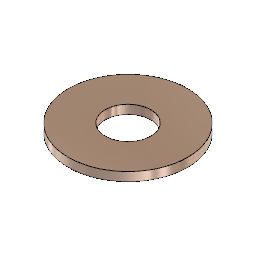
SHVFeedthroughFilterWithPulseLine_LEGEND60 (Autodesk Fusion 360 archive; units mm, degrees)
design "Washer"
Autodesk Fusion 360 part; units mm, degrees
sketch "Sketch1" plane through (0, 0, 0) normal (0, 0, 1) x (1, 0, 0)
  circle A0 centre (0, 0) radius 8.5
  circle A1 centre (0, 0) radius 3.2385
  dimension "d1" = 17
  dimension "d2" = 6.477
  constraint coincident A0.centre A1.centre
  measures "d1" diameter of A0
  measures "d2" diameter of A1
extrude "Extrude1" add sketch "Sketch1" along normal blind 1.27
sketch "Sketch2" plane through (0, 0, 0) normal (0, 0, -1) x (1, 0, 0)
  arc A0 (-2.7777, 8.0333) -> (2.7777, 8.0333) centre (0, 15) ccw
  circle A1 centre (0, 0) radius 8.5
  line L0 (0, -1.75) -> (0, -22.5)
  dimension "d6" = 15
  dimension "d10" = 7.5
  constraint coincident A0.end A1
  constraint coincident A0.start A1
  constraint coincident A0.centre L0
  measures "d6" distance of A1.centre A0.centre
  measures "d10" radius of A0
extrude "Extrude2" [rolled back] taper angle 0
pattern_circular "C-Pattern1" [rolled back] total angle 360

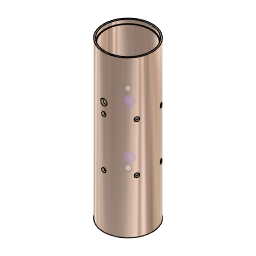
design "OuterTube"
Autodesk Fusion 360 part; units mm, degrees
sketch "Sketch1" plane through (0, 0, 0) normal (0, 0, 1) x (1, 0, 0)
  circle A0 centre (0, 0) radius 9.525
  circle A1 centre (0, 0) radius 8.7122
  dimension "d1" = 19.05
  dimension "d2" = 0.8128
  constraint coincident A0.centre A1.centre
  constraint concentric A0 A1
  measures "d1" diameter of A0
  measures "d2" distance of A0 A1
extrude "Extrude1" add sketch "Sketch1" along normal blind 76
sketch "Sketch2" plane through (0, 0, 0) normal (1, 0, 0) x (0, 1, 0)
  line L0 (0, 1.75) -> (0, 22.5)
  point P0 (0, 8)
  dimension "d8" = 8
  constraint coincident P0 L0
  measures "d8" distance of origin P0
hole "Hole1" at (0, 0, 8) direction (-1, 0, 0) diameter 2.3813 depth 30 tip angle 118
sketch "Sketch3" plane through (0, 0, 0) normal (0, 1, 0) x (1, 0, 0)
  point P0 (0, -36)
  dimension "d9" = 36
  measures "d9" distance of origin P0
hole "Hole2" at (0, 0, 36) direction (0, -1, 0) diameter 1.5875 depth 20 tip angle 118
pattern_circular "C-Pattern1" count 6 over 360 about axis through (0, 0, 1.75) along (0, 0, 1) of "Hole2"
sketch "Sketch4" plane through (0, 0, 0) normal (0, 0, -1) x (1, 0, 0)
  circle A0 centre (0, 0) radius 8.7122
  circle A1 centre (0, 0) radius 9.525
  circle A2 centre (0, 0) radius 9
  dimension "d15" = 18
  constraint coincident A0.centre A1.centre
  measures "d15" diameter of A2
extrude "Extrude2" cut sketch "Sketch4" against normal blind 1.5 contours A2
sketch "Sketch5" plane through (0, 0, 76) normal (0, 0, 1) x (-1, 0, 0)
  circle A0 centre (0, 0) radius 8.7122
  circle A1 centre (0, 0) radius 9.525
  circle A2 centre (0, 0) radius 9
  dimension "d18" = 18
  constraint concentric A0 A2
  measures "d18" diameter of A2
extrude "Extrude3" cut sketch "Sketch5" against normal blind 1.5 contours A2
sketch "Sketch7" plane through (0, 0, 0) normal (0, 1, 0) x (1, 0, 0)
  line L0 (9.525, 0) -> (-9.525, 0)
  line L1 (-9.525, -76) -> (9.525, -76)
  point P0 (0, -55)
  dimension "d42" = 21
  measures "d42" distance of P0 L1
hole "Hole4" at (0, 0, 55) direction (0, -1, 0) diameter 1.5875 end through all
pattern_circular "C-Pattern2" count 6 over 360 about axis through (0, 0, 1.75) along (0, 0, 1) of "Hole4"
sketch "Sketch8" plane through (0, 0, 0) normal (0, 0, -1) x (1, 0, 0)
  circle A0 centre (0, 0) radius 9
  circle A1 centre (0, 0) radius 9.525
  line L0 (7.064, 5.5449) -> (8.334, 3.3451)
  line L1 (8.334, 3.3451) -> (-7.064, -5.5449)
  line L2 (-7.064, -5.5449) -> (-8.334, -3.3451)
  line L3 (-8.334, -3.3451) -> (7.064, 5.5449)
  line L4 (1.75, 0) -> (22.5, 0)
  line L5 (0, -1.75) -> (0, -22.5)
  line L6 (-0.635, 1.0999) -> (0, 0)
  line L7 (0, 0) -> (7.699, 4.445)
  point P0 (-0.635, 1.0999)
  point P1 (7.699, 4.445)
  dimension "d31" = 17.78
  dimension "d32" = 2.54
  dimension "d38" = 30
  constraint coincident A0.centre A1.centre
  constraint perpendicular L0 L3
  constraint perpendicular L1 L2
  constraint parallel L1 L3
  constraint midpoint L3 P0
  constraint midpoint L0 P1
  constraint coincident P0 L6.start
  constraint coincident P1 L7.end
  constraint perpendicular L3 L6
  constraint perpendicular L0 L7
  measures "d31" distance of L0.start L2.end
  measures "d32" distance of L0.start L0.end
  measures "d38" angle of L1 L4
sketch "Sketch9" plane through (0, 0, 0) normal (0, 0, 1) x (1, 0, 0)
  circle A0 centre (0, 0) radius 9.525
extrude "Extrude5" cut sketch "Sketch9" along normal blind 15
sketch "Sketch10" plane through (0, 0, 0) normal (0, 1, 0) x (1, 0, 0)
  spline S0 degree 3 poles (0.7937, -36) (0.7937, -35.9003) (0.7738, -35.794) (0.6928, -35.5984) (0.6317, -35.5092) (0.4908, -35.3683) (0.4016, -35.3072) (0.206, -35.2262) (0.0997, -35.2062) (-0.0997, -35.2062) (-0.206, -35.2262) (-0.4016, -35.3072) (-0.4908, -35.3683) (-0.6317, -35.5092) (-0.6928, -35.5984) (-0.7738, -35.794) (-0.7937, -35.9003) (-0.7937, -36.0997) (-0.7738, -36.206) (-0.6928, -36.4016) (-0.6317, -36.4908) (-0.4908, -36.6317) (-0.4016, -36.6928) (-0.206, -36.7738) (-0.0997, -36.7938) (0.0997, -36.7938) (0.206, -36.7738) (0.4016, -36.6928) (0.4908, -36.6317) (0.6317, -36.4908) (0.6928, -36.4016) (0.7738, -36.206) (0.7937, -36.0997) (0.7937, -36) knots 0 0 0 0 0.029914 0.029914 0.059829 0.059829 0.089743 0.089743 0.119658 0.119658 0.149572 0.149572 0.179486 0.179486 0.209401 0.209401 0.239315 0.239315 0.26923 0.26923 0.299144 0.299144 0.329058 0.329058 0.358973 0.358973 0.388887 0.388887 0.418801 0.418801 0.448716 0.448716 0.47863 0.47863 0.47863 0.47863
  spline S1 degree 3 poles (0.7937, -55) (0.7937, -54.9003) (0.7738, -54.794) (0.6928, -54.5984) (0.6317, -54.5092) (0.4908, -54.3683) (0.4016, -54.3072) (0.206, -54.2262) (0.0997, -54.2062) (-0.0997, -54.2063) (-0.206, -54.2262) (-0.4016, -54.3072) (-0.4908, -54.3683) (-0.6317, -54.5092) (-0.6928, -54.5984) (-0.7738, -54.794) (-0.7937, -54.9003) (-0.7937, -55.0997) (-0.7738, -55.206) (-0.6928, -55.4016) (-0.6317, -55.4908) (-0.4908, -55.6317) (-0.4016, -55.6928) (-0.206, -55.7738) (-0.0997, -55.7937) (0.0997, -55.7937) (0.206, -55.7738) (0.4016, -55.6928) (0.4908, -55.6317) (0.6317, -55.4908) (0.6928, -55.4016) (0.7738, -55.206) (0.7937, -55.0997) (0.7937, -55) knots 0 0 0 0 0.029914 0.029914 0.059829 0.059829 0.089743 0.089743 0.119658 0.119658 0.149572 0.149572 0.179486 0.179486 0.209401 0.209401 0.239315 0.239315 0.26923 0.26923 0.299144 0.299144 0.329058 0.329058 0.358973 0.358973 0.388887 0.388887 0.418801 0.418801 0.448716 0.448716 0.47863 0.47863 0.47863 0.47863
  point P0 (0, -32)
  point P1 (0, -59)
  point P2 (0.7937, -55)
  point P3 (0.7937, -36)
  dimension "d43" = 4
  dimension "d44" = 4
  measures "d43" distance of P1 S1.start
  measures "d44" vertical distance of P0 P3
hole "Hole5" at (0, 0, 59) direction (0, -1, 0) diameter 2.3813 end through all
hole "Hole6" at (0, 0, 32) direction (0, 1, 0) diameter 2.3813 end through all
equation "d6 = 3 in / 32"
equation "d11 = 1 in / 16"
equation "d27 = 1 in / 16"
equation "d46 = 3 in / 32"
equation "d49 = 3 in / 32"

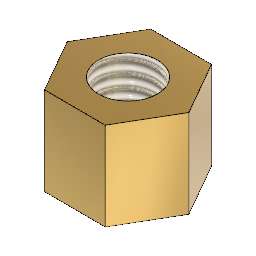
design "CapacitorArrayCenter"
Autodesk Fusion 360 part; units mm, degrees
sketch "Sketch1" plane through (0, 0, 0) normal (0, 0, 1) x (1, 0, 0)
  line L0 (1.7454, 2.9923) -> (-1.7187, 3.0077)
  line L1 (-1.7187, 3.0077) -> (-3.4641, 0.0154)
  line L2 (-3.4641, 0.0154) -> (-1.7454, -2.9923)
  line L3 (-1.7454, -2.9923) -> (1.7187, -3.0077)
  line L4 (1.7187, -3.0077) -> (3.4641, -0.0154)
  line L5 (3.4641, -0.0154) -> (1.7454, 2.9923)
  dimension "d1" = 6
  measures "d1" distance of L0 L3
extrude "Extrude1" add sketch "Sketch1" along normal mid plane 5
sketch "Sketch2" plane through (0, 0, 2.5) normal (0, 0, 1) x (-1, 0, 0)
  line L0 (-3.4641, 0.0154) -> (-1.7454, -2.9923)
  line L1 (-1.7454, -2.9923) -> (1.7187, -3.0077)
  line L2 (1.7187, -3.0077) -> (3.4641, -0.0154)
  line L3 (3.4641, -0.0154) -> (1.7454, 2.9923)
  line L4 (1.7454, 2.9923) -> (-1.7187, 3.0077)
  line L5 (-1.7187, 3.0077) -> (-3.4641, 0.0154)
hole "Hole1" at (0, 0, 2.5) direction (0, 0, -1) diameter 3.332 end through all
thread "Thread1" "ISO Metric profile 4.0 M4x0.7 6H" major diameter 4.1095 minor diameter 3.332 pitch 0.7 angle 60 resizes the face on face at (0.083, -1.6639, 0.8333)

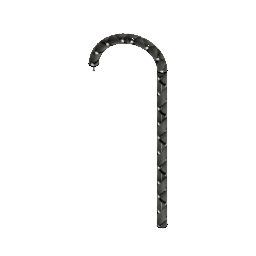
design "LMR-100"
Autodesk Fusion 360 part; units mm, degrees
sketch "Sketch2" plane through (0, 0, 0) normal (0, 0, 1) x (-1, 0, 0)
  circle A0 centre (-10.92, 0) radius 1.055
  line L0 (-10.92, 0) -> (0, 7.8)
  line L1 (-5.46, 3.9) -> (-2.6743, 0)
  dimension "d28" = 2.11
  dimension "d29" = 7.8
  dimension "d31" = 10.92
  constraint coincident A0.centre L0.start
  constraint midpoint L0 L1.start
  constraint perpendicular L0 L1
  constraint vertical origin L0.end
  constraint horizontal origin A0.centre
  constraint horizontal origin L1.end
  measures "d28" diameter of A0
  measures "d29" distance of origin L0.end
  measures "d31" distance of origin A0.centre
revolve "Revolve1" add sketch "Sketch2" angle 180 about axis through (5.46, -3.9, 0) along (0.581238, -0.813733, 0) makes body 1
sketch "Sketch3" plane through (0, 0, 0) normal (0, 0, -1) x (1, 0, 0)
  circle A0 centre (10.92, 0) radius 1.055
extrude "Extrude2" add sketch "Sketch3" along normal blind 36.8 bodies 1
sketch "Sketch6" plane through (0, 0, 0) normal (0, 0, -1) x (1, 0, 0)
  circle A0 centre (0, 7.8) radius 0.25
  circle A1 centre (0, 7.8) radius 1.055
  dimension "d25" = 0.5
  constraint coincident A0.centre A1.centre
  measures "d25" diameter of A0
extrude "Extrude3" add sketch "Sketch6" along normal blind 1.6 separate body contours A0 makes body 2
equation "d7 = 50 mm - 13.2 mm"
equation "d31 = ( 0.75 in + 2.79 mm ) / 2"
equation "d17 = 74 mm - 10.8 mm"

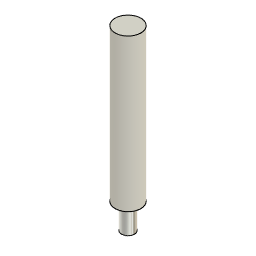
design "LEGENDCable"
Autodesk Fusion 360 part; units mm, degrees
sketch "Sketch1" plane through (0, 0, 0) normal (0, 0, 1) x (1, 0, 0)
  circle A0 centre (0, 0) radius 1.27
  dimension "d1" = 2.54
  constraint coincident A0.centre origin
  measures "d1" diameter of A0
extrude "Extrude1" add sketch "Sketch1" along normal blind 5 makes body 1
sketch "Sketch2" plane through (0, 0, 5) normal (0, 0, 1) x (-1, 0, 0)
  circle A0 centre (0, 0) radius 1.27
  circle A1 centre (0, 0) radius 2.54
  dimension "d4" = 5.08
  constraint coincident A0.centre A1.centre
  measures "d4" diameter of A1
extrude "Extrude2" add sketch "Sketch2" along normal blind 30 separate body contours A0 | A1 makes body 2

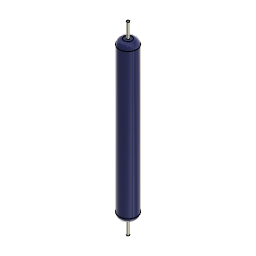
design "MOX1125-22"
Autodesk Fusion 360 part; units mm, degrees
sketch "Sketch1" plane through (0, 0, 0) normal (0, 0, 1) x (1, 0, 0)
  circle A0 centre (0, 0) radius 1.78
  dimension "d1" = 3.56
  constraint coincident A0.centre origin
  measures "d1" diameter of A0
extrude "Extrude1" add sketch "Sketch1" along normal mid plane 31 makes body 1
sketch "Sketch2" plane through (0, 0, 15.5) normal (0, 0, 1) x (-1, 0, 0)
  circle A0 centre (0, 0) radius 1.78
  circle A1 centre (0, 0) radius 0.254
  dimension "d4" = 0.508
  constraint concentric A0 A1
  measures "d4" diameter of A1
extrude "Extrude2" add sketch "Sketch2" along normal blind 3 separate body contours A1 makes body 2
mirror "Mirror1" about plane through (0, 0, 0) normal (0, 0, 1) of "Extrude2" makes body 3
fillet "Fillet1" radius 1 2 edges at (-1.6595, -0.6437, 15.5) (-1.6595, 0.6437, -15.5) on bodies 1

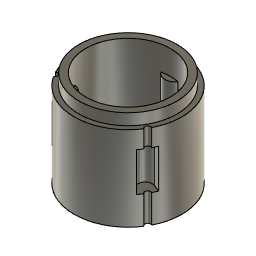
design "TubeInsulator"
Autodesk Fusion 360 part; units mm, degrees
sketch "Sketch1" plane through (0, 0, 0) normal (0, 0, 1) x (1, 0, 0)
  circle A0 centre (0, 0) radius 9.575
  dimension "d36" = 19.15
  constraint coincident A0.centre origin
  measures "d36" diameter of A0
extrude "Extrude1" add sketch "Sketch1" along normal blind 15
sketch "Sketch2" plane through (0, 0, 0) normal (0, 0, -1) x (1, 0, 0)
  circle A0 centre (0, 0) radius 9.575
hole "Hole1" at (0, 0, 0) direction (0, 0, 1) diameter 15 end through all
hole "Hole2" at (0, 0, 0) direction (0, 0, 1) diameter 17.55 depth 1.8 tip angle 118
sketch "Sketch3" plane through (0, 0, 0) normal (0, 1, 0) x (1, 0, 0)
  circle A0 centre (0, -7.5) radius 7.5
  line L0 (-9.575, -15) -> (9.575, -15)
  line L1 (-9.575, 0) -> (9.575, 0)
  line L2 (9.575, 0) -> (-9.575, 0)
  constraint vertical origin A0.centre
  constraint tangent A0 L0
  constraint tangent A0 L2
hole "Hole3" [suppressed]
thread "Thread1" [suppressed]
sketch "Sketch4" plane through (0, 0, 15) normal (0, 0, 1) x (-1, 0, 0)
  circle A0 centre (0, 0) radius 7.5
  circle A1 centre (0, 0) radius 9.575
  circle A2 centre (0, 0) radius 7.5
  circle A3 centre (0, 0) radius 8.7122
  dimension "d15" = 17.4244
  constraint concentric A0 A3
  measures "d15" diameter of A3
extrude "Extrude2" add sketch "Sketch4" along normal blind 2 contours A3
sketch "Sketch5" plane through (0, 0, 0) normal (0, 0, 1) x (1, 0, 0)
  circle A0 centre (0, 9.55) radius 0.775
  circle A1 centre (0, 0) radius 8.775
  constraint tangent A0 A1
hole "Hole4" at (0, 9.55, 0) direction (0, 0, 1) diameter 1 end through all
ref_plane "WorkPlane1" through (0, 0, 7.5) normal (0, 0, -1) x (-1, 0, 0)
sketch "Sketch6" plane through (0, -0.0066, 7.5) normal (0, 0, -1) x (1, 0, 0)
  circle A0 centre (0, -8.3316) radius 1.25
  arc A1 (0.4999, -9.5685) -> (-0.4999, -9.5685) centre (0, -0.0066) ccw
  line L0 (-1.2359, -8.144) -> (-1.4375, -9.473)
  line L1 (1.2359, -8.144) -> (1.4375, -9.473)
  arc A2 (-1.4375, -9.473) -> (1.4375, -9.473) centre (0, -0.0066) ccw
  dimension "d22" = 2.5
  constraint tangent A0 A1
  constraint vertical origin A0.centre
  constraint coincident A0 L0.start
  constraint coincident A1 L0.end
  constraint coincident A0 L1.start
  constraint coincident A1 L1.end
  constraint tangent A0 L1
  constraint tangent A0 L0
  constraint coincident origin L0
  constraint coincident origin L1
  constraint coincident A1.centre A2.centre
  measures "d22" diameter of A0
sketch "Sketch7" plane through (0, -0.0066, 7.5) normal (0, 0, -1) x (1, 0, 0)
  circle A0 centre (0, -8.3316) radius 1.8028
  circle A1 centre (0, -8.3316) radius 1.25
  arc A2 (0.4999, -9.5685) -> (-0.4999, -9.5685) centre (0, -9.5566) ccw
  arc A3 (-1.4375, -9.473) -> (1.4375, -9.473) centre (0, -0.0066) ccw
  constraint concentric A0 A1
extrude "Extrude4" add sketch "Sketch7" along normal blind 3.3 and the other way blind 5.2 contours A0 A1 A2 A3 | A1 A2 picked at (0.0221, -7.7427)
extrude "Extrude5" cut sketch "Sketch6" along normal blind 2.5 and the other way blind 4.4 contours A0 | A0 A1 L1 A2 | A0 A1 L0 A2
pattern_circular "C-Pattern1" count 3 over 360 about axis through (0, 0, 1.75) along (0, 0, 1) of "Hole4", "Extrude4", "Extrude5"
hole "Hole5" at (0, 0, 0) direction (0, 0, 1) diameter 15.1 depth 4.2 tip angle 118
